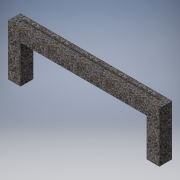
# Autodesk Inventor part: RailsMini
Saved by Autodesk Inventor 2016 (Build 200138000, 138)
## iProperties
Created: 2015-08-15
Part Number: RailsMini
Material: Concrete
Document SubType Name: Modeling
Designer: myhome
Density: 2.40731 g/cm^3
Appearance: Exposed Aggregate - Coarse
Mass: 43331.6 g
Surface Area: 7400 cm^2
Volume: 18000 cm^3
Author: myhome
Autodesk Inventor part; units mm, degrees
ref_plane "YZ Plane" through (0, 0, 0) normal (1, 0, 0) x (0, 1, 0)
ref_plane "XZ Plane" through (0, 0, 0) normal (0, 1, 0) x (-1, 0, 0)
ref_plane "XY Plane" through (0, 0, 0) normal (0, 0, 1) x (1, 0, 0)
sketch "Sketch1" plane through (0, 0, 0) normal (0, 0, 1) x (1, 0, 0)
  line L0 (0, 0) -> (0, 400)
  line L1 (0, 400) -> (1200, 400)
  line L2 (1100, 300) -> (100, 300)
  line L3 (100, 300) -> (100, 0)
  line L4 (100, 0) -> (0, 0)
  line L5 (1100, 300) -> (1100, 0)
  line L6 (1100, 0) -> (1200, 0)
  line L7 (1200, 0) -> (1200, 400)
  dimension "d0" = 400
  dimension "d1" = 1200
  dimension "d5" = 1000
  dimension "d6" = 300
  dimension "d7" = 100
  dimension "d10" = 300
  dimension "d11" = 100
  dimension "d12" = 400
  constraints: 16 end point, 3 perpendicular, 2 vertical
  measures "d0" distance of L0.start L0.end
  measures "d1" distance of L0.end L1.end
  measures "d5" distance of L2.start L2.end
  measures "d6" distance of L2.end L3.end
  measures "d7" distance of L3.end L0.start
  measures "d10" distance of L2.start L5.end
  measures "d11" distance of L5.end L6.end
  measures "d12" distance of L6.end L1.end
extrude "Extrusion1" add sketch "Sketch1" against normal blind 100
sketch "Sketch2" plane through (0, 400, 0) normal (0, 1, 0) x (1, 0, 0)
  line L0 (0, 100) -> (1200, 100) projected
  line L1 (0, 100) -> (50, 100)
  line L2 (0, 0) -> (1200, 0) construction
  line L3 (50, 0) -> (0, 0)
  line L4 (1200, 0) -> (1150, 0)
  line L5 (50, 100) -> (50, 65)
  line L6 (50, 65) -> (50, 35)
  line L7 (50, 35) -> (50, 0)
  line L8 (1150, 100) -> (1150, 65)
  line L9 (1150, 65) -> (1150, 35)
  line L10 (1150, 35) -> (1150, 0)
  line L11 (50, 65) -> (1150, 65)
  line L12 (1150, 65) -> (1150, 35)
  line L13 (1150, 35) -> (50, 35)
  line L14 (50, 35) -> (50, 65)
  dimension "d13" = 50
  dimension "d14" = 50
  dimension "d15" = 35
  dimension "d16" = 30
  dimension "d17" = 35
  dimension "d18" = 35
  dimension "d19" = 30
  dimension "d20" = 35
  constraints: 26 end point, 5 point on line, 2 collinear, 2 parallel, 2 perpendicular, 2 vertical, 1 horizontal
  measures "d13" distance of L0.start L1.end
  measures "d14" distance of L2.end L4.end
  measures "d15" distance of L1.end L5.end
  measures "d16" distance of L5.end L6.end
  measures "d17" distance of L6.end L3.start
  measures "d18" distance of L8.start L8.end
  measures "d19" distance of L8.end L9.end
  measures "d20" distance of L9.end L4.end
extrude "Extrusion2" cut sketch "Sketch2" against normal blind 8 contours L11 L9 L13 L6
body "Solid1"
